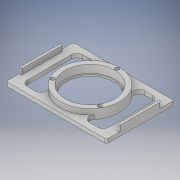
# Autodesk Inventor part: Sensor Halterung63
Saved by Autodesk Inventor 2017 (Build 210142000, 142)
## iProperties
Part Number: Sensor Halterung63
Material: Generisch
Document SubType Name: Modeling
Designer: Harald.Noeske
Density: 1 g/cm^3
Appearance: Vorgabe
Author: Harald.Noeske
Autodesk Inventor part; units mm, degrees
ref_plane "YZ Plane" through (0, 0, 0) normal (1, 0, 0) x (0, 1, 0)
ref_plane "XZ Plane" through (0, 0, 0) normal (0, 1, 0) x (-1, 0, 0)
ref_plane "XY Plane" through (0, 0, 0) normal (0, 0, 1) x (1, 0, 0)
sketch "Skizze1" plane through (0, 0, 0) normal (0, 0, 1) x (1, 0, 0)
  line L0 (0, 0) -> (127.5, 0)
  line L1 (127.5, 0) -> (127.5, -85.5)
  line L2 (127.5, -85.5) -> (0, -85.5)
  line L3 (0, -85.5) -> (0, 0)
  dimension "d0" = 127.5
  dimension "d1" = 85.5
  constraints: 8 end point, 2 parallel, 1 horizontal, 1 perpendicular
  measures "d0" distance of L1.end L2.end
  measures "d1" distance of L0.end L1.end
extrude "Extrusion1" add sketch "Skizze1" along normal blind 5
sketch "Skizze2" plane through (0, 0, 5) normal (0, 0, 1) x (1, 0, 0)
  line L0 (0, -16.25) -> (3, -16.25)
  line L1 (3, -16.25) -> (3, -69.25)
  line L2 (3, -69.25) -> (0, -69.25)
  line L3 (0, -69.25) -> (0, -16.25)
  line L4 (63.75, 42.9175) -> (63.75, -147.2432)
  line L5 (127.5, -85.5) -> (127.5, 0) projected
  line L6 (127.5, -16.25) -> (124.5, -16.25)
  line L7 (124.5, -16.25) -> (124.5, -69.25)
  line L8 (124.5, -69.25) -> (127.5, -69.25)
  line L9 (127.5, -69.25) -> (127.5, -16.25)
  point P0 (0, 0)
  dimension "d4" = 3
  dimension "d5" = 53
  dimension "d6" = 16.25
  dimension "d7" = 63.75
  constraints: 18 end point, 4 symmetric about line, 2 parallel, 1 horizontal, 1 perpendicular, 1 vertical
  measures "d4" distance of L1.end L2.end
  measures "d5" distance of L0.end L1.end
  measures "d6" distance of L0.start point (0, 0)
  measures "d7" distance between parallel lines of L4 L5
extrude "Extrusion2" add sketch "Skizze2" along normal blind 7
fillet "Rundung1" radius 2 4 edges at (0, 0, 2.5) (127.5, 0, 2.5) (127.5, -85.5, 2.5) (0, -85.5, 2.5)
fillet "Rundung2" radius 1.5 8 edges at (3, -69.25, 8.5) (0, -69.25, 8.5) (3, -16.25, 8.5) (0, -16.25, 8.5) (124.5, -16.25, 8.5) (127.5, -16.25, 8.5) (124.5, -69.25, 8.5) (127.5, -69.25, 8.5)
sketch "Skizze3" plane through (0, 0, 5) normal (0, 0, 1) x (1, 0, 0)
  circle A0 centre (63.75, -42.75) radius 30
  line L0 (0, -67.75) -> (0, -83.5) projected
  point P0 (0, 0)
  dimension "d12" = 60
  dimension "d13" = 63.75
  dimension "d14" = 42.75
  constraints: 1 centre point
  measures "d12" diameter of A0
  measures "d13" distance from line of A0.centre L0
  measures "d14" vertical distance of point (0, 0) A0.centre
extrude "Extrusion3" cut sketch "Skizze3" against normal blind 10
hole "Bohrung1" at (63.75, -42.75, 5) direction (0, 0, -1) diameter 63 depth 3
sketch "Skizze4" plane through (0, 0, 0) normal (0, 0, -1) x (-1, 0, 0)
  line L0 (-125.5, -85.5) -> (-2, -85.5) projected
  line L1 (0, -83.5) -> (0, -2) projected
  line L2 (-12, -77.75) -> (-50.2871, -77.75)
  line L3 (-50.2871, -7.75) -> (-12, -7.75)
  line L4 (-12, -7.75) -> (-12, -77.75)
  line L5 (-63.75, -42.75) -> (-63.75, -99.3052)
  line L6 (-115.5, -77.75) -> (-77.2129, -77.75)
  line L7 (-77.2129, -7.75) -> (-115.5, -7.75)
  line L8 (-115.5, -7.75) -> (-115.5, -77.75)
  arc A0 (-50.2871, -77.75) -> (-50.2871, -7.75) centre (-63.75, -42.75) ccw
  arc A1 (-77.2129, -7.75) -> (-77.2129, -77.75) centre (-63.75, -42.75) ccw
  arc A2 (-50.2871, -77.75) -> (-50.2871, -7.75) centre (-63.75, -42.75) ccw
  arc A3 (-77.2129, -7.75) -> (-77.2129, -77.75) centre (-63.75, -42.75) ccw
  point P0 (0, 0)
  dimension "d27" = 42.75
  dimension "d28" = 63.75
  dimension "d29" = 12
  dimension "d30" = 70
  dimension "d31" = 7.75
  constraints: 14 end point, 8 point on circle, 4 centre point, 4 symmetric about line, 1 horizontal, 1 parallel, 1 vertical
  measures "d27" distance from line of L0 L5.start
  measures "d28" distance from line of L5.start L1
  measures "d29" distance between parallel lines of L4 L1
  measures "d30" distance of L3.end L2.start
  measures "d31" distance between parallel lines of L0 L2
extrude "Extrusion4" cut sketch "Skizze4" against normal blind 10
fillet "Rundung3" radius 7 4 edges at (50.2871, -77.75, 2.5) (77.2129, -77.75, 2.5) (50.2871, -7.75, 2.5) (77.2129, -7.75, 2.5)
fillet "Rundung4" radius 7 4 edges at (12, -77.75, 2.5) (115.5, -77.75, 2.5) (12, -7.75, 2.5) (115.5, -7.75, 2.5)
sketch "Skizze5" plane through (0, 0, 5) normal (0, 0, 1) x (1, 0, 0)
  circle A0 centre (63.75, -42.75) radius 31.5
  circle A1 centre (63.75, -42.75) radius 37.5
  line L0 (125.5, 0) -> (2, 0) projected
  point P0 (0, 0)
  dimension "d36" = 63
  dimension "d37" = 75
  dimension "d38" = 42.75
  dimension "d39" = 63.75
  constraints: 2 centre point, 1 coincident
  measures "d36" diameter of A0
  measures "d37" diameter of A1
  measures "d38" distance from line of A0.centre L0
  measures "d39" horizontal distance of point (0, 0) A0.centre
extrude "Extrusion5" add sketch "Skizze5" along normal blind 7
sketch "Skizze6" plane through (63.75, -42.75, 12) normal (0, 0, 1) x (1, 0, 0)
  circle A0 centre (-0.0001, 34.5) radius 2.525
  circle A1 centre (0, 0) radius 31.5 projected
  point P0 (-63.75, 42.75)
  dimension "d42" = 5.05
  dimension "d43" = 34.5
  constraints: 1 centre point
  measures "d42" diameter of A0
  measures "d43" distance of A1.centre A0.centre
extrude "Extrusion6" cut sketch "Skizze6" against normal blind 2.1 contours A0
pattern_circular "Runde Anordnung1" count 3 over 360 about axis through (63.75, -42.75, 3.5) along (0, 0, 1) of "Extrusion6"
